Autodesk Inventor part; units mm, degrees
(part 3 of 4)
  line L513 (170.4618, 600.3596) -> (170.0567, 600.3596)
  line L514 (170.0567, 600.3596) -> (170.0567, 603.4076)
  line L515 (170.0567, 603.4076) -> (170.4618, 603.4076)
  line L516 (170.4618, 603.4076) -> (170.4618, 602.2121)
  line L517 (170.4618, 602.2121) -> (171.8647, 602.2121)
  line L518 (171.8647, 602.2121) -> (171.8647, 603.4076)
  line L519 (171.8647, 603.4076) -> (172.2698, 603.4076)
  line L520 (172.2698, 603.4076) -> (172.2698, 600.3596)
  line L521 (174.7621, 601.4069) -> (174.399, 601.4069)
  line L522 (174.399, 601.4069) -> (174.399, 600.3596)
  line L523 (174.399, 600.3596) -> (174.0063, 600.3596)
  line L524 (174.0063, 600.3596) -> (174.0063, 601.4069)
  line L525 (174.0063, 601.4069) -> (172.6601, 601.4069)
  line L526 (172.6601, 601.4069) -> (172.6601, 601.8366)
  line L527 (172.6601, 601.8366) -> (174.0235, 603.4076)
  line L528 (174.0235, 603.4076) -> (174.399, 603.4076)
  line L529 (174.399, 603.4076) -> (174.399, 601.7354)
  line L530 (174.399, 601.7354) -> (174.7621, 601.7354)
  line L531 (174.7621, 601.7354) -> (174.7621, 601.4069)
  line L532 (174.0063, 601.7354) -> (174.0063, 602.9259)
  line L533 (174.0063, 602.9259) -> (172.9812, 601.7354)
  line L534 (172.9812, 601.7354) -> (174.0063, 601.7354)
  line L535 (176.9678, 600.3596) -> (175.0881, 600.3596)
  line L536 (175.0881, 600.3596) -> (175.0881, 600.7918)
  spline S514 degree 2 poles (175.0881, 600.7918) (175.2907, 600.982) (175.6513, 601.3352) (175.8242, 601.5254) knots 0 0 0 1 2 2 2
  spline S515 degree 2 poles (175.8242, 601.5254) (176.1725, 601.9083) (176.4269, 602.3677) (176.4269, 602.6122) knots 0 0 0 1 2 2 2
  spline S516 degree 2 poles (176.4269, 602.6122) (176.4269, 602.7407) (176.3478, 602.9333) (176.2762, 602.9951) knots 0 0 0 1 2 2 2
  spline S517 degree 2 poles (176.2762, 602.9951) (176.2046, 603.0568) (176.0168, 603.1186) (175.9032, 603.1186) knots 0 0 0 1 2 2 2
  spline S518 degree 2 poles (175.9032, 603.1186) (175.7945, 603.1186) (175.5722, 603.0642) (175.471, 603.0222) knots 0 0 0 1 2 2 2
  spline S519 degree 2 poles (175.471, 603.0222) (175.3845, 602.9877) (175.224, 602.8889) (175.1746, 602.8543) knots 0 0 0 1 2 2 2
  line L537 (175.1746, 602.8543) -> (175.1523, 602.8543)
  line L538 (175.1523, 602.8543) -> (175.1523, 603.289)
  spline S520 degree 2 poles (175.1523, 603.289) (175.2783, 603.3508) (175.7303, 603.4718) (175.9329, 603.4718) knots 0 0 0 1 2 2 2
  spline S521 degree 2 poles (175.9329, 603.4718) (176.3602, 603.4718) (176.8418, 603.0198) (176.8418, 602.6344) knots 0 0 0 1 2 2 2
  spline S522 degree 2 poles (176.8418, 602.6344) (176.8418, 602.4541) (176.7578, 602.1528) (176.6837, 602.0244) knots 0 0 0 1 2 2 2
  spline S523 degree 2 poles (176.6837, 602.0244) (176.6096, 601.891) (176.3948, 601.6292) (176.2762, 601.5032) knots 0 0 0 1 2 2 2
  spline S524 degree 2 poles (176.2762, 601.5032) (176.0835, 601.2932) (175.6118, 600.8437) (175.471, 600.7128) knots 0 0 0 1 2 2 2
  line L539 (175.471, 600.7128) -> (176.9678, 600.7128)
  line L540 (176.9678, 600.7128) -> (176.9678, 600.3596)
  spline S525 degree 2 poles (179.3884, 602.4887) (179.3884, 602.2911) (179.2476, 601.9354) (179.1217, 601.8119) knots 0 0 0 1 2 2 2
  spline S526 degree 2 poles (179.1217, 601.8119) (178.9636, 601.6563) (178.5363, 601.4958) (178.2102, 601.4958) knots 0 0 0 1 2 2 2
  line L541 (178.2102, 601.4958) -> (177.8669, 601.4958)
  line L542 (177.8669, 601.4958) -> (177.8669, 600.3596)
  line L543 (177.8669, 600.3596) -> (177.4618, 600.3596)
  line L544 (177.4618, 600.3596) -> (177.4618, 603.4076)
  line L545 (177.4618, 603.4076) -> (178.2275, 603.4076)
  spline S527 degree 2 poles (178.2275, 603.4076) (178.4992, 603.4076) (178.8796, 603.3186) (179.0253, 603.2174) knots 0 0 0 1 2 2 2
  spline S528 degree 2 poles (179.0253, 603.2174) (179.1958, 603.1013) (179.3884, 602.7431) (179.3884, 602.4887) knots 0 0 0 1 2 2 2
  spline S529 degree 2 poles (178.966, 602.4764) (178.966, 602.6344) (178.8574, 602.8666) (178.7462, 602.9407) knots 0 0 0 1 2 2 2
  spline S530 degree 2 poles (178.7462, 602.9407) (178.6499, 603.005) (178.393, 603.0568) (178.2028, 603.0568) knots 0 0 0 1 2 2 2
  line L546 (178.2028, 603.0568) -> (177.8669, 603.0568)
  line L547 (177.8669, 603.0568) -> (177.8669, 601.8416)
  line L548 (177.8669, 601.8416) -> (178.1435, 601.8416)
  spline S531 degree 2 poles (178.1435, 601.8416) (178.3905, 601.8416) (178.6943, 601.9206) (178.7931, 602.0244) knots 0 0 0 1 2 2 2
  spline S532 degree 2 poles (178.7931, 602.0244) (178.8845, 602.1157) (178.966, 602.3306) (178.966, 602.4764) knots 0 0 0 1 2 2 2
  line L549 (181.9968, 600.3596) -> (181.4706, 600.3596)
  line L550 (181.4706, 600.3596) -> (180.3567, 601.7774)
  line L551 (180.3567, 601.7774) -> (180.1788, 601.5773)
  line L552 (180.1788, 601.5773) -> (180.1788, 600.3596)
  line L553 (180.1788, 600.3596) -> (179.7737, 600.3596)
  line L554 (179.7737, 600.3596) -> (179.7737, 603.4076)
  line L555 (179.7737, 603.4076) -> (180.1788, 603.4076)
  line L556 (180.1788, 603.4076) -> (180.1788, 602.0071)
  line L557 (180.1788, 602.0071) -> (181.4286, 603.4076)
  line L558 (181.4286, 603.4076) -> (181.9227, 603.4076)
  line L559 (181.9227, 603.4076) -> (180.6605, 602.0466)
  line L560 (180.6605, 602.0466) -> (181.9968, 600.3596)
  line L561 (183.4195, 603.5434) -> (182.2265, 599.6976)
  line L562 (182.2265, 599.6976) -> (181.8807, 599.6976)
  line L563 (181.8807, 599.6976) -> (183.0687, 603.5434)
  line L564 (183.0687, 603.5434) -> (183.4195, 603.5434)
  line L565 (185.025, 602.2343) -> (185.0052, 602.2343)
  spline S533 degree 2 poles (185.0052, 602.2343) (184.9608, 602.2467) (184.8644, 602.2516) (184.7978, 602.2516) knots 0 0 0 1 2 2 2
  spline S534 degree 2 poles (184.7978, 602.2516) (184.6421, 602.2516) (184.3359, 602.1157) (184.1975, 601.9824) knots 0 0 0 1 2 2 2
  line L566 (184.1975, 601.9824) -> (184.1975, 600.3596)
  line L567 (184.1975, 600.3596) -> (183.8122, 600.3596)
  line L568 (183.8122, 600.3596) -> (183.8122, 602.6468)
  line L569 (183.8122, 602.6468) -> (184.1975, 602.6468)
  line L570 (184.1975, 602.6468) -> (184.1975, 602.3059)
  spline S535 degree 2 poles (184.1975, 602.3059) (184.4075, 602.4937) (184.7212, 602.6468) (184.8694, 602.6468) knots 0 0 0 1 2 2 2
  spline S536 degree 2 poles (184.8694, 602.6468) (184.9287, 602.6468) (184.9879, 602.6419) (185.025, 602.6344) knots 0 0 0 1 2 2 2
  line L571 (185.025, 602.6344) -> (185.025, 602.2343)
  spline S537 degree 2 poles (186.3168, 600.3077) (185.7685, 600.3077) (185.1658, 600.9227) (185.1658, 601.4908) knots 0 0 0 1 2 2 2
  spline S538 degree 2 poles (185.1658, 601.4908) (185.1658, 602.0491) (185.7512, 602.711) (186.223, 602.711) knots 0 0 0 1 2 2 2
  spline S539 degree 2 poles (186.223, 602.711) (186.4354, 602.711) (186.7639, 602.5875) (186.8849, 602.4566) knots 0 0 0 1 2 2 2
  spline S540 degree 2 poles (186.8849, 602.4566) (187.0084, 602.3257) (187.1393, 601.9478) (187.1393, 601.6736) knots 0 0 0 1 2 2 2
  line L572 (187.1393, 601.6736) -> (187.1393, 601.4637)
  line L573 (187.1393, 601.4637) -> (185.556, 601.4637)
  spline S541 degree 2 poles (185.556, 601.4637) (185.556, 601.066) (185.9562, 600.6436) (186.3119, 600.6436) knots 0 0 0 1 2 2 2
  spline S542 degree 2 poles (186.3119, 600.6436) (186.4378, 600.6436) (186.6824, 600.7004) (186.7812, 600.7449) knots 0 0 0 1 2 2 2
  spline S543 degree 2 poles (186.7812, 600.7449) (186.8849, 600.7943) (187.0282, 600.8807) (187.0751, 600.9203) knots 0 0 0 1 2 2 2
  line L574 (187.0751, 600.9203) -> (187.0973, 600.9203)
  line L575 (187.0973, 600.9203) -> (187.0973, 600.5004)
  spline S544 degree 2 poles (187.0973, 600.5004) (187.0306, 600.4732) (186.8281, 600.3941) (186.7491, 600.3719) knots 0 0 0 1 2 2 2
  spline S545 degree 2 poles (186.7491, 600.3719) (186.6379, 600.3398) (186.4551, 600.3077) (186.3168, 600.3077) knots 0 0 0 1 2 2 2
  spline S546 degree 2 poles (186.7639, 601.7576) (186.7589, 601.9132) (186.6947, 602.1404) (186.633, 602.217) knots 0 0 0 1 2 2 2
  spline S547 degree 2 poles (186.633, 602.217) (186.5663, 602.3035) (186.3563, 602.3949) (186.2007, 602.3949) knots 0 0 0 1 2 2 2
  spline S548 degree 2 poles (186.2007, 602.3949) (186.0476, 602.3949) (185.8327, 602.3035) (185.7438, 602.2145) knots 0 0 0 1 2 2 2
  spline S549 degree 2 poles (185.7438, 602.2145) (185.6573, 602.1232) (185.5684, 601.9033) (185.556, 601.7576) knots 0 0 0 1 2 2 2
  line L576 (185.556, 601.7576) -> (186.7639, 601.7576)
  line L577 (188.7325, 603.1729) -> (188.7127, 603.1729)
  spline S550 degree 2 poles (188.7127, 603.1729) (188.6609, 603.1927) (188.4682, 603.2273) (188.3916, 603.2273) knots 0 0 0 1 2 2 2
  spline S551 degree 2 poles (188.3916, 603.2273) (188.1496, 603.2273) (187.9421, 603.0099) (187.9421, 602.7234) knots 0 0 0 1 2 2 2
  line L578 (187.9421, 602.7234) -> (187.9421, 602.6468)
  line L579 (187.9421, 602.6468) -> (188.5793, 602.6468)
  line L580 (188.5793, 602.6468) -> (188.5793, 602.3282)
  line L581 (188.5793, 602.3282) -> (187.9544, 602.3282)
  line L582 (187.9544, 602.3282) -> (187.9544, 600.3596)
  line L583 (187.9544, 600.3596) -> (187.5691, 600.3596)
  line L584 (187.5691, 600.3596) -> (187.5691, 602.3282)
  line L585 (187.5691, 602.3282) -> (187.3098, 602.3282)
  line L586 (187.3098, 602.3282) -> (187.3098, 602.6468)
  line L587 (187.3098, 602.6468) -> (187.5691, 602.6468)
  line L588 (187.5691, 602.6468) -> (187.5691, 602.7234)
  spline S552 degree 2 poles (187.5691, 602.7234) (187.5691, 603.1334) (187.9668, 603.5632) (188.3373, 603.5632) knots 0 0 0 1 2 2 2
  spline S553 degree 2 poles (188.3373, 603.5632) (188.4435, 603.5632) (188.6485, 603.5409) (188.7325, 603.5261) knots 0 0 0 1 2 2 2
  line L589 (188.7325, 603.5261) -> (188.7325, 603.1729)
  line L590 (191.2396, 601.1006) -> (188.977, 601.1006)
  line L591 (188.977, 601.1006) -> (188.977, 601.4291)
  line L592 (188.977, 601.4291) -> (191.2396, 601.4291)
  line L593 (191.2396, 601.4291) -> (191.2396, 601.1006)
  line L594 (191.2396, 601.9601) -> (188.977, 601.9601)
  line L595 (188.977, 601.9601) -> (188.977, 602.2886)
  line L596 (188.977, 602.2886) -> (191.2396, 602.2886)
  line L597 (191.2396, 602.2886) -> (191.2396, 601.9601)
  spline S554 degree 2 poles (192.5314, 600.3052) (192.3017, 600.3052) (191.904, 600.4287) (191.7731, 600.4979) knots 0 0 0 1 2 2 2
  line L598 (191.7731, 600.4979) -> (191.7731, 600.9301)
  line L599 (191.7731, 600.9301) -> (191.7928, 600.9301)
  spline S555 degree 2 poles (191.7928, 600.9301) (191.8422, 600.8906) (191.9756, 600.7968) (192.0868, 600.7449) knots 0 0 0 1 2 2 2
  spline S556 degree 2 poles (192.0868, 600.7449) (192.1831, 600.698) (192.4202, 600.6288) (192.5462, 600.6288) knots 0 0 0 1 2 2 2
  spline S557 degree 2 poles (192.5462, 600.6288) (192.6376, 600.6288) (192.8475, 600.6708) (192.8969, 600.7054) knots 0 0 0 1 2 2 2
  spline S558 degree 2 poles (192.8969, 600.7054) (192.9686, 600.7523) (193.0328, 600.8585) (193.0328, 600.9672) knots 0 0 0 1 2 2 2
  spline S559 degree 2 poles (193.0328, 600.9672) (193.0328, 601.103) (192.8846, 601.2438) (192.6944, 601.2908) knots 0 0 0 1 2 2 2
  spline S560 degree 2 poles (192.6944, 601.2908) (192.6203, 601.3081) (192.3832, 601.3575) (192.2819, 601.3846) knots 0 0 0 1 2 2 2
  spline S561 degree 2 poles (192.2819, 601.3846) (192.0201, 601.4612) (191.783, 601.7774) (191.783, 602.0021) knots 0 0 0 1 2 2 2
  spline S562 degree 2 poles (191.783, 602.0021) (191.783, 602.3133) (192.2498, 602.7011) (192.6351, 602.7011) knots 0 0 0 1 2 2 2
  spline S563 degree 2 poles (192.6351, 602.7011) (192.8253, 602.7011) (193.2106, 602.6073) (193.3415, 602.5356) knots 0 0 0 1 2 2 2
  line L600 (193.3415, 602.5356) -> (193.3415, 602.1232)
  line L601 (193.3415, 602.1232) -> (193.3218, 602.1232)
  spline S564 degree 2 poles (193.3218, 602.1232) (193.1736, 602.2417) (192.813, 602.3776) (192.6277, 602.3776) knots 0 0 0 1 2 2 2
  spline S565 degree 2 poles (192.6277, 602.3776) (192.4375, 602.3776) (192.1757, 602.217) (192.1757, 602.0565) knots 0 0 0 1 2 2 2
  spline S566 degree 2 poles (192.1757, 602.0565) (192.1757, 601.9107) (192.3313, 601.7699) (192.5042, 601.7255) knots 0 0 0 1 2 2 2
  spline S567 degree 2 poles (192.5042, 601.7255) (192.5882, 601.7033) (192.8006, 601.6588) (192.9167, 601.6316) knots 0 0 0 1 2 2 2
  spline S568 degree 2 poles (192.9167, 601.6316) (193.1686, 601.5674) (193.4255, 601.2735) (193.4255, 601.0191) knots 0 0 0 1 2 2 2
  spline S569 degree 2 poles (193.4255, 601.0191) (193.4255, 600.8709) (193.3094, 600.609) (193.1958, 600.5127) knots 0 0 0 1 2 2 2
  spline S570 degree 2 poles (193.1958, 600.5127) (193.0748, 600.4114) (192.766, 600.3052) (192.5314, 600.3052) knots 0 0 0 1 2 2 2
  line L602 (194.9964, 602.2343) -> (194.9767, 602.2343)
  spline S571 degree 2 poles (194.9767, 602.2343) (194.9322, 602.2467) (194.8359, 602.2516) (194.7692, 602.2516) knots 0 0 0 1 2 2 2
  spline S572 degree 2 poles (194.7692, 602.2516) (194.6136, 602.2516) (194.3073, 602.1157) (194.169, 601.9824) knots 0 0 0 1 2 2 2
  line L603 (194.169, 601.9824) -> (194.169, 600.3596)
  line L604 (194.169, 600.3596) -> (193.7837, 600.3596)
  line L605 (193.7837, 600.3596) -> (193.7837, 602.6468)
  line L606 (193.7837, 602.6468) -> (194.169, 602.6468)
  line L607 (194.169, 602.6468) -> (194.169, 602.3059)
  spline S573 degree 2 poles (194.169, 602.3059) (194.3789, 602.4937) (194.6926, 602.6468) (194.8408, 602.6468) knots 0 0 0 1 2 2 2
  spline S574 degree 2 poles (194.8408, 602.6468) (194.9001, 602.6468) (194.9594, 602.6419) (194.9964, 602.6344) knots 0 0 0 1 2 2 2
  line L608 (194.9964, 602.6344) -> (194.9964, 602.2343)
  line L609 (197.3356, 599.747) -> (194.9841, 599.747)
  line L610 (194.9841, 599.747) -> (194.9841, 600.0113)
  line L611 (194.9841, 600.0113) -> (197.3356, 600.0113)
  line L612 (197.3356, 600.0113) -> (197.3356, 599.747)
  line L613 (199.2523, 600.3596) -> (197.7653, 600.3596)
  line L614 (197.7653, 600.3596) -> (197.7653, 600.6708)
  line L615 (197.7653, 600.6708) -> (198.3186, 600.6708)
  line L616 (198.3186, 600.6708) -> (198.3186, 602.7135)
  line L617 (198.3186, 602.7135) -> (197.7653, 602.7135)
  line L618 (197.7653, 602.7135) -> (197.7653, 602.9926)
  spline S575 degree 2 poles (197.7653, 602.9926) (198.079, 602.9926) (198.3754, 603.1704) (198.3952, 603.4174) knots 0 0 0 1 2 2 2
  line L619 (198.3952, 603.4174) -> (198.7114, 603.4174)
  line L620 (198.7114, 603.4174) -> (198.7114, 600.6708)
  line L621 (198.7114, 600.6708) -> (199.2523, 600.6708)
  line L622 (199.2523, 600.6708) -> (199.2523, 600.3596)
  line L623 (201.91, 599.747) -> (199.5586, 599.747)
  line L624 (199.5586, 599.747) -> (199.5586, 600.0113)
  line L625 (199.5586, 600.0113) -> (201.91, 600.0113)
  line L626 (201.91, 600.0113) -> (201.91, 599.747)
  spline S576 degree 2 poles (202.9227, 603.1186) (202.8116, 603.1186) (202.5917, 603.0642) (202.4855, 603.0222) knots 0 0 0 1 2 2 2
  spline S577 degree 2 poles (202.4855, 603.0222) (202.3867, 602.9803) (202.241, 602.8913) (202.1842, 602.8518) knots 0 0 0 1 2 2 2
  line L627 (202.1842, 602.8518) -> (202.1595, 602.8518)
  line L628 (202.1595, 602.8518) -> (202.1595, 603.2841)
  spline S578 degree 2 poles (202.1595, 603.2841) (202.2929, 603.3557) (202.7498, 603.4718) (202.9548, 603.4718) knots 0 0 0 1 2 2 2
  spline S579 degree 2 poles (202.9548, 603.4718) (203.1623, 603.4718) (203.4711, 603.3878) (203.597, 603.2989) knots 0 0 0 1 2 2 2
  spline S580 degree 2 poles (203.597, 603.2989) (203.7304, 603.2026) (203.8687, 602.9234) (203.8687, 602.7357) knots 0 0 0 1 2 2 2
  spline S581 degree 2 poles (203.8687, 602.7357) (203.8687, 602.4838) (203.5378, 602.1034) (203.3056, 602.054) knots 0 0 0 1 2 2 2
  line L629 (203.3056, 602.054) -> (203.3056, 602.0244)
  spline S582 degree 2 poles (203.3056, 602.0244) (203.4019, 602.0046) (203.6217, 601.9157) (203.7156, 601.8268) knots 0 0 0 1 2 2 2
  spline S583 degree 2 poles (203.7156, 601.8268) (203.8095, 601.7403) (203.928, 601.4637) (203.928, 601.2636) knots 0 0 0 1 2 2 2
  spline S584 degree 2 poles (203.928, 601.2636) (203.928, 601.0586) (203.7872, 600.7103) (203.6588, 600.5769) knots 0 0 0 1 2 2 2
  spline S585 degree 2 poles (203.6588, 600.5769) (203.5254, 600.4386) (203.1475, 600.2953) (202.9079, 600.2953) knots 0 0 0 1 2 2 2
  spline S586 degree 2 poles (202.9079, 600.2953) (202.6782, 600.2953) (202.2287, 600.4065) (202.0755, 600.4831) knots 0 0 0 1 2 2 2
  line L630 (202.0755, 600.4831) -> (202.0755, 600.9153)
  line L631 (202.0755, 600.9153) -> (202.1052, 600.9153)
  spline S587 degree 2 poles (202.1052, 600.9153) (202.2336, 600.8215) (202.6683, 600.6486) (202.8832, 600.6486) knots 0 0 0 1 2 2 2
  spline S588 degree 2 poles (202.8832, 600.6486) (203.0092, 600.6486) (203.2611, 600.7276) (203.3451, 600.819) knots 0 0 0 1 2 2 2
  spline S589 degree 2 poles (203.3451, 600.819) (203.4266, 600.9104) (203.5131, 601.1277) (203.5131, 601.2932) knots 0 0 0 1 2 2 2
  spline S590 degree 2 poles (203.5131, 601.2932) (203.5131, 601.4587) (203.4167, 601.6736) (203.3303, 601.7354) knots 0 0 0 1 2 2 2
  spline S591 degree 2 poles (203.3303, 601.7354) (203.2438, 601.7971) (203.0092, 601.844) (202.8709, 601.844) knots 0 0 0 1 2 2 2
  line L632 (202.8709, 601.844) -> (202.698, 601.844)
  line L633 (202.698, 601.844) -> (202.698, 602.1824)
  line L634 (202.698, 602.1824) -> (202.8338, 602.1824)
  spline S592 degree 2 poles (202.8338, 602.1824) (203.108, 602.1824) (203.4538, 602.4443) (203.4538, 602.6937) knots 0 0 0 1 2 2 2
  spline S593 degree 2 poles (203.4538, 602.6937) (203.4538, 602.8098) (203.3649, 602.9753) (203.2932, 603.0247) knots 0 0 0 1 2 2 2
  spline S594 degree 2 poles (203.2932, 603.0247) (203.2167, 603.0766) (203.0289, 603.1186) (202.9227, 603.1186) knots 0 0 0 1 2 2 2
  spline S595 degree 2 poles (206.03, 602.6913) (206.03, 602.4912) (205.8966, 602.1775) (205.7855, 602.0589) knots 0 0 0 1 2 2 2
  spline S596 degree 2 poles (205.7855, 602.0589) (205.6768, 601.9404) (205.3952, 601.7403) (205.2396, 601.6464) knots 0 0 0 1 2 2 2
  line L635 (205.2396, 601.6464) -> (205.2396, 601.1796)
  line L636 (205.2396, 601.1796) -> (204.874, 601.1796)
  line L637 (204.874, 601.1796) -> (204.874, 601.8045)
  spline S597 degree 2 poles (204.874, 601.8045) (204.9877, 601.8737) (205.2939, 602.0663) (205.3804, 602.1503) knots 0 0 0 1 2 2 2
  spline S598 degree 2 poles (205.3804, 602.1503) (205.4891, 602.2565) (205.6126, 602.5035) (205.6126, 602.6616) knots 0 0 0 1 2 2 2
  spline S599 degree 2 poles (205.6126, 602.6616) (205.6126, 602.8913) (205.3211, 603.1186) (205.0889, 603.1186) knots 0 0 0 1 2 2 2
  spline S600 degree 2 poles (205.0889, 603.1186) (204.8839, 603.1186) (204.5233, 602.9827) (204.4097, 602.9086) knots 0 0 0 1 2 2 2
  line L638 (204.4097, 602.9086) -> (204.3875, 602.9086)
  line L639 (204.3875, 602.9086) -> (204.3875, 603.3261)
  spline S601 degree 2 poles (204.3875, 603.3261) (204.5233, 603.3804) (204.9407, 603.4693) (205.1285, 603.4693) knots 0 0 0 1 2 2 2
  spline S602 degree 2 poles (205.1285, 603.4693) (205.5484, 603.4693) (206.03, 603.042) (206.03, 602.6913) knots 0 0 0 1 2 2 2
  line L640 (205.2717, 600.3596) -> (204.8568, 600.3596)
  line L641 (204.8568, 600.3596) -> (204.8568, 600.7918)
  line L642 (204.8568, 600.7918) -> (205.2717, 600.7918)
  line L643 (205.2717, 600.7918) -> (205.2717, 600.3596)
  line L644 (206.8229, 600.3596) -> (206.4376, 600.3596)
  line L645 (206.4376, 600.3596) -> (206.4376, 602.6468)
  line L646 (206.4376, 602.6468) -> (206.8229, 602.6468)
  line L647 (206.8229, 602.6468) -> (206.8229, 600.3596)
  line L648 (206.8501, 603.0272) -> (206.4129, 603.0272)
  line L649 (206.4129, 603.0272) -> (206.4129, 603.4273)
  line L650 (206.4129, 603.4273) -> (206.8501, 603.4273)
  line L651 (206.8501, 603.4273) -> (206.8501, 603.0272)
  spline S603 degree 2 poles (208.3815, 600.3077) (207.8331, 600.3077) (207.2304, 600.9227) (207.2304, 601.4908) knots 0 0 0 1 2 2 2
  spline S604 degree 2 poles (207.2304, 601.4908) (207.2304, 602.0491) (207.8158, 602.711) (208.2876, 602.711) knots 0 0 0 1 2 2 2
  spline S605 degree 2 poles (208.2876, 602.711) (208.5, 602.711) (208.8285, 602.5875) (208.9496, 602.4566) knots 0 0 0 1 2 2 2
  spline S606 degree 2 poles (208.9496, 602.4566) (209.0731, 602.3257) (209.204, 601.9478) (209.204, 601.6736) knots 0 0 0 1 2 2 2
  line L652 (209.204, 601.6736) -> (209.204, 601.4637)
  line L653 (209.204, 601.4637) -> (207.6207, 601.4637)
  spline S607 degree 2 poles (207.6207, 601.4637) (207.6207, 601.066) (208.0208, 600.6436) (208.3765, 600.6436) knots 0 0 0 1 2 2 2
  spline S608 degree 2 poles (208.3765, 600.6436) (208.5025, 600.6436) (208.747, 600.7004) (208.8458, 600.7449) knots 0 0 0 1 2 2 2
  spline S609 degree 2 poles (208.8458, 600.7449) (208.9496, 600.7943) (209.0928, 600.8807) (209.1398, 600.9203) knots 0 0 0 1 2 2 2
  line L654 (209.1398, 600.9203) -> (209.162, 600.9203)
  line L655 (209.162, 600.9203) -> (209.162, 600.5004)
  spline S610 degree 2 poles (209.162, 600.5004) (209.0953, 600.4732) (208.8928, 600.3941) (208.8137, 600.3719) knots 0 0 0 1 2 2 2
  spline S611 degree 2 poles (208.8137, 600.3719) (208.7026, 600.3398) (208.5198, 600.3077) (208.3815, 600.3077) knots 0 0 0 1 2 2 2
  spline S612 degree 2 poles (208.8285, 601.7576) (208.8236, 601.9132) (208.7594, 602.1404) (208.6976, 602.217) knots 0 0 0 1 2 2 2
  spline S613 degree 2 poles (208.6976, 602.217) (208.6309, 602.3035) (208.421, 602.3949) (208.2654, 602.3949) knots 0 0 0 1 2 2 2
  spline S614 degree 2 poles (208.2654, 602.3949) (208.1122, 602.3949) (207.8973, 602.3035) (207.8084, 602.2145) knots 0 0 0 1 2 2 2
  spline S615 degree 2 poles (207.8084, 602.2145) (207.722, 602.1232) (207.6331, 601.9033) (207.6207, 601.7576) knots 0 0 0 1 2 2 2
  line L656 (207.6207, 601.7576) -> (208.8285, 601.7576)
  line L657 (211.9704, 601.1006) -> (209.7079, 601.1006)
  line L658 (209.7079, 601.1006) -> (209.7079, 601.4291)
  line L659 (209.7079, 601.4291) -> (211.9704, 601.4291)
  line L660 (211.9704, 601.4291) -> (211.9704, 601.1006)
  line L661 (211.9704, 601.9601) -> (209.7079, 601.9601)
  line L662 (209.7079, 601.9601) -> (209.7079, 602.2886)
  line L663 (209.7079, 602.2886) -> (211.9704, 602.2886)
  line L664 (211.9704, 602.2886) -> (211.9704, 601.9601)
  spline S616 degree 2 poles (213.7389, 600.2953) (213.4697, 600.2953) (213.0696, 600.4361) (212.9288, 600.5769) knots 0 0 0 1 2 2 2
  spline S617 degree 2 poles (212.9288, 600.5769) (212.7682, 600.735) (212.6373, 601.1796) (212.6373, 601.5057) knots 0 0 0 1 2 2 2
  line L665 (212.6373, 601.5057) -> (212.6373, 603.4076)
  line L666 (212.6373, 603.4076) -> (213.0424, 603.4076)
  line L667 (213.0424, 603.4076) -> (213.0424, 601.5057)
  spline S618 degree 2 poles (213.0424, 601.5057) (213.0424, 601.2932) (213.0967, 601.0067) (213.1733, 600.8906) knots 0 0 0 1 2 2 2
  spline S619 degree 2 poles (213.1733, 600.8906) (213.2548, 600.7671) (213.5364, 600.6411) (213.7389, 600.6411) knots 0 0 0 1 2 2 2
  spline S620 degree 2 poles (213.7389, 600.6411) (213.9291, 600.6411) (214.2255, 600.7671) (214.307, 600.8906) knots 0 0 0 1 2 2 2
  spline S621 degree 2 poles (214.307, 600.8906) (214.3836, 601.0067) (214.4379, 601.2908) (214.4379, 601.4958) knots 0 0 0 1 2 2 2
  line L668 (214.4379, 601.4958) -> (214.4379, 603.4076)
  line L669 (214.4379, 603.4076) -> (214.843, 603.4076)
  line L670 (214.843, 603.4076) -> (214.843, 601.5057)
  spline S622 degree 2 poles (214.843, 601.5057) (214.843, 601.187) (214.7146, 600.7325) (214.5516, 600.5769) knots 0 0 0 1 2 2 2
  spline S623 degree 2 poles (214.5516, 600.5769) (214.4058, 600.4337) (214.0205, 600.2953) (213.7389, 600.2953) knots 0 0 0 1 2 2 2
  line L671 (216.1348, 600.3596) -> (216.1348, 603.0469)
  line L672 (216.1348, 603.0469) -> (215.1123, 603.0469)
  line L673 (215.1123, 603.0469) -> (215.1123, 603.4076)
  line L674 (215.1123, 603.4076) -> (217.5625, 603.4076)
  line L675 (217.5625, 603.4076) -> (217.5625, 603.0469)
  line L676 (217.5625, 603.0469) -> (216.5399, 603.0469)
  line L677 (216.5399, 603.0469) -> (216.5399, 600.3596)
  line L678 (216.5399, 600.3596) -> (216.1348, 600.3596)
  line L679 (219.6941, 603.0469) -> (218.2764, 603.0469)
  line L680 (218.2764, 603.0469) -> (218.2764, 602.1874)
  line L681 (218.2764, 602.1874) -> (219.6349, 602.1874)
  line L682 (219.6349, 602.1874) -> (219.6349, 601.8268)
  line L683 (219.6349, 601.8268) -> (218.2764, 601.8268)
  line L684 (218.2764, 601.8268) -> (218.2764, 600.3596)
  line L685 (218.2764, 600.3596) -> (217.8713, 600.3596)
  line L686 (217.8713, 600.3596) -> (217.8713, 603.4076)
  line L687 (217.8713, 603.4076) -> (219.6941, 603.4076)
  line L688 (219.6941, 603.4076) -> (219.6941, 603.0469)
  spline S624 degree 2 poles (220.8921, 600.2904) (220.6649, 600.2904) (220.2919, 600.4263) (220.161, 600.5522) knots 0 0 0 1 2 2 2
  spline S625 degree 2 poles (220.161, 600.5522) (220.0325, 600.6757) (219.8992, 601.0116) (219.8992, 601.2018) knots 0 0 0 1 2 2 2
  spline S626 degree 2 poles (219.8992, 601.2018) (219.8992, 601.4488) (220.1634, 601.8638) (220.4154, 601.9873) knots 0 0 0 1 2 2 2
  line L689 (220.4154, 601.9873) -> (220.4154, 601.9997)
  spline S627 degree 2 poles (220.4154, 601.9997) (220.1906, 602.1306) (219.9733, 602.4418) (219.9733, 602.674) knots 0 0 0 1 2 2 2
  spline S628 degree 2 poles (219.9733, 602.674) (219.9733, 603.0173) (220.492, 603.4767) (220.8921, 603.4767) knots 0 0 0 1 2 2 2
  spline S629 degree 2 poles (220.8921, 603.4767) (221.3071, 603.4767) (221.8085, 603.042) (221.8085, 602.7011) knots 0 0 0 1 2 2 2
  spline S630 degree 2 poles (221.8085, 602.7011) (221.8085, 602.4961) (221.5689, 602.096) (221.3441, 601.9824) knots 0 0 0 1 2 2 2
  line L690 (221.3441, 601.9824) -> (221.3441, 601.97)
  spline S631 degree 2 poles (221.3441, 601.97) (221.6109, 601.8465) (221.885, 601.4908) (221.885, 601.2093) knots 0 0 0 1 2 2 2
  spline S632 degree 2 poles (221.885, 601.2093) (221.885, 600.819) (221.3169, 600.2904) (220.8921, 600.2904) knots 0 0 0 1 2 2 2
  spline S633 degree 2 poles (221.4651, 601.1697) (221.4651, 601.3575) (221.3169, 601.5798) (221.107, 601.6934) knots 0 0 0 1 2 2 2
  spline S634 degree 2 poles (221.107, 601.6934) (221.0378, 601.7329) (220.8056, 601.8243) (220.6599, 601.8836) knots 0 0 0 1 2 2 2
  spline S635 degree 2 poles (220.6599, 601.8836) (220.492, 601.7724) (220.3116, 601.4414) (220.3116, 601.2315) knots 0 0 0 1 2 2 2
  spline S636 degree 2 poles (220.3116, 601.2315) (220.3116, 600.9548) (220.6451, 600.5942) (220.897, 600.5942) knots 0 0 0 1 2 2 2
  spline S637 degree 2 poles (220.897, 600.5942) (221.1539, 600.5942) (221.4651, 600.903) (221.4651, 601.1697) knots 0 0 0 1 2 2 2
  spline S638 degree 2 poles (221.4083, 602.6962) (221.4083, 602.9012) (221.1342, 603.1754) (220.8896, 603.1754) knots 0 0 0 1 2 2 2
  spline S639 degree 2 poles (220.8896, 603.1754) (220.6673, 603.1754) (220.3833, 602.9309) (220.3833, 602.7209) knots 0 0 0 1 2 2 2
  spline S640 degree 2 poles (220.3833, 602.7209) (220.3833, 602.5702) (220.529, 602.3603) (220.6747, 602.2763) knots 0 0 0 1 2 2 2
  spline S641 degree 2 poles (220.6747, 602.2763) (220.7365, 602.2417) (220.9983, 602.1207) (221.1045, 602.0861) knots 0 0 0 1 2 2 2
  spline S642 degree 2 poles (221.1045, 602.0861) (221.2824, 602.222) (221.4083, 602.5109) (221.4083, 602.6962) knots 0 0 0 1 2 2 2
  line L691 (224.9923, 600.3596) -> (224.4687, 600.3596)
  line L692 (224.4687, 600.3596) -> (224.0512, 600.7968)
  spline S643 degree 2 poles (224.0512, 600.7968) (223.8438, 600.53) (223.4041, 600.2953) (223.125, 600.2953) knots 0 0 0 1 2 2 2
  spline S644 degree 2 poles (223.125, 600.2953) (222.7125, 600.2953) (222.174, 600.7943) (222.174, 601.1969) knots 0 0 0 1 2 2 2
  spline S645 degree 2 poles (222.174, 601.1969) (222.174, 601.3723) (222.2728, 601.6464) (222.3543, 601.7576) knots 0 0 0 1 2 2 2
  spline S646 degree 2 poles (222.3543, 601.7576) (222.4334, 601.8638) (222.6433, 602.0268) (222.7372, 602.0861) knots 0 0 0 1 2 2 2
  spline S647 degree 2 poles (222.7372, 602.0861) (222.5322, 602.2244) (222.3272, 602.5332) (222.3272, 602.7654) knots 0 0 0 1 2 2 2
  spline S648 degree 2 poles (222.3272, 602.7654) (222.3272, 602.9111) (222.4433, 603.1581) (222.5371, 603.252) knots 0 0 0 1 2 2 2
  spline S649 degree 2 poles (222.5371, 603.252) (222.6359, 603.3483) (222.9496, 603.4718) (223.1349, 603.4718) knots 0 0 0 1 2 2 2
  spline S650 degree 2 poles (223.1349, 603.4718) (223.4757, 603.4718) (223.9055, 603.1136) (223.9055, 602.8395) knots 0 0 0 1 2 2 2
  spline S651 degree 2 poles (223.9055, 602.8395) (223.9055, 602.7382) (223.8536, 602.5233) (223.787, 602.4245) knots 0 0 0 1 2 2 2
  spline S652 degree 2 poles (223.787, 602.4245) (223.7178, 602.3232) (223.5004, 602.1479) (223.3177, 602.0812) knots 0 0 0 1 2 2 2
  line L693 (223.3177, 602.0812) -> (224.0364, 601.3402)
  spline S653 degree 2 poles (224.0364, 601.3402) (224.0636, 601.5081) (224.0759, 601.9033) (224.0759, 602.222) knots 0 0 0 1 2 2 2
  line L694 (224.0759, 602.222) -> (224.4761, 602.222)
  line L695 (224.4761, 602.222) -> (224.4761, 602.0244)
  spline S654 degree 2 poles (224.4761, 602.0244) (224.4761, 601.8292) (224.3773, 601.3352) (224.2612, 601.1129) knots 0 0 0 1 2 2 2
  line L696 (224.2612, 601.1129) -> (224.9923, 600.3596)
  line L697 (223.8734, 600.9771) -> (222.9323, 601.9404)
  spline S655 degree 2 poles (222.9323, 601.9404) (222.8829, 601.9083) (222.7817, 601.8169) (222.7199, 601.728) knots 0 0 0 1 2 2 2
  spline S656 degree 2 poles (222.7199, 601.728) (222.6705, 601.6563) (222.5964, 601.4241) (222.5964, 601.2957) knots 0 0 0 1 2 2 2
  spline S657 degree 2 poles (222.5964, 601.2957) (222.5964, 601.0042) (222.9422, 600.6288) (223.2361, 600.6288) knots 0 0 0 1 2 2 2
  spline S658 degree 2 poles (223.2361, 600.6288) (223.4313, 600.6288) (223.745, 600.7943) (223.8734, 600.9771) knots 0 0 0 1 2 2 2
  spline S659 degree 2 poles (223.125, 602.2269) (223.2386, 602.2664) (223.3893, 602.3973) (223.4313, 602.4739) knots 0 0 0 1 2 2 2
  spline S660 degree 2 poles (223.4313, 602.4739) (223.4683, 602.5455) (223.5054, 602.7061) (223.5054, 602.7999) knots 0 0 0 1 2 2 2
  spline S661 degree 2 poles (223.5054, 602.7999) (223.5054, 602.9975) (223.2732, 603.2149) (223.1201, 603.2149) knots 0 0 0 1 2 2 2
  spline S662 degree 2 poles (223.1201, 603.2149) (222.9373, 603.2149) (222.7273, 602.9679) (222.7273, 602.7851) knots 0 0 0 1 2 2 2
  spline S663 degree 2 poles (222.7273, 602.7851) (222.7273, 602.7036) (222.757, 602.585) (222.8064, 602.5085) knots 0 0 0 1 2 2 2
  spline S664 degree 2 poles (222.8064, 602.5085) (222.8508, 602.4443) (223.004, 602.301) (223.125, 602.2269) knots 0 0 0 1 2 2 2
  line L698 (226.8967, 599.5173) -> (226.5114, 599.5173)
  line L699 (226.5114, 599.5173) -> (226.5114, 600.609)
  spline S665 degree 2 poles (226.5114, 600.609) (226.3434, 600.4559) (226.0248, 600.3151) (225.8297, 600.3151) knots 0 0 0 1 2 2 2
  spline S666 degree 2 poles (225.8297, 600.3151) (225.4419, 600.3151) (224.98, 600.94) (224.98, 601.4958) knots 0 0 0 1 2 2 2
  spline S667 degree 2 poles (224.98, 601.4958) (224.98, 601.7922) (225.1405, 602.2442) (225.2739, 602.3973) knots 0 0 0 1 2 2 2
  spline S668 degree 2 poles (225.2739, 602.3973) (225.4023, 602.548) (225.7531, 602.711) (225.9433, 602.711) knots 0 0 0 1 2 2 2
  spline S669 degree 2 poles (225.9433, 602.711) (226.1187, 602.711) (226.3755, 602.6295) (226.5114, 602.548) knots 0 0 0 1 2 2 2
  line L700 (226.5114, 602.548) -> (226.5361, 602.6468)
  line L701 (226.5361, 602.6468) -> (226.8967, 602.6468)
  line L702 (226.8967, 602.6468) -> (226.8967, 599.5173)
  line L703 (226.5114, 600.9326) -> (226.5114, 602.2368)
  spline S670 degree 2 poles (226.5114, 602.2368) (226.3657, 602.3084) (226.1384, 602.3652) (226.0075, 602.3652) knots 0 0 0 1 2 2 2
  spline S671 degree 2 poles (226.0075, 602.3652) (225.7037, 602.3652) (225.3776, 601.9256) (225.3776, 601.5155) knots 0 0 0 1 2 2 2
  spline S672 degree 2 poles (225.3776, 601.5155) (225.3776, 601.1129) (225.6395, 600.6807) (225.9161, 600.6807) knots 0 0 0 1 2 2 2
  spline S673 degree 2 poles (225.9161, 600.6807) (226.0767, 600.6807) (226.3829, 600.819) (226.5114, 600.9326) knots 0 0 0 1 2 2 2
  line L704 (227.8477, 600.3596) -> (227.4623, 600.3596)
  line L705 (227.4623, 600.3596) -> (227.4623, 602.6468)
  line L706 (227.4623, 602.6468) -> (227.8477, 602.6468)
  line L707 (227.8477, 602.6468) -> (227.8477, 600.3596)
  line L708 (227.8748, 603.0272) -> (227.4376, 603.0272)
  line L709 (227.4376, 603.0272) -> (227.4376, 603.4273)
  line L710 (227.4376, 603.4273) -> (227.8748, 603.4273)
  line L711 (227.8748, 603.4273) -> (227.8748, 603.0272)
  line L712 (230.1719, 600.3596) -> (229.7866, 600.3596)
  line L713 (229.7866, 600.3596) -> (229.7866, 600.5917)
  spline S674 degree 2 poles (229.7866, 600.5917) (229.6977, 600.5176) (229.5668, 600.4188) (229.4779, 600.3769) knots 0 0 0 1 2 2 2
  spline S675 degree 2 poles (229.4779, 600.3769) (229.3964, 600.3373) (229.221, 600.2953) (229.1049, 600.2953) knots 0 0 0 1 2 2 2
  spline S676 degree 2 poles (229.1049, 600.2953) (228.9172, 600.2953) (228.601, 600.451) (228.4899, 600.6016) knots 0 0 0 1 2 2 2
  spline S677 degree 2 poles (228.4899, 600.6016) (228.3787, 600.7523) (228.2552, 601.1969) (228.2552, 601.4859) knots 0 0 0 1 2 2 2
  spline S678 degree 2 poles (228.2552, 601.4859) (228.2552, 601.7872) (228.4108, 602.2269) (228.5467, 602.3924) knots 0 0 0 1 2 2 2
  spline S679 degree 2 poles (228.5467, 602.3924) (228.6727, 602.5406) (229.0259, 602.711) (229.221, 602.711) knots 0 0 0 1 2 2 2
  spline S680 degree 2 poles (229.221, 602.711) (229.3914, 602.711) (229.6458, 602.6344) (229.7866, 602.5554) knots 0 0 0 1 2 2 2
  line L714 (229.7866, 602.5554) -> (229.7866, 603.5434)
  line L715 (229.7866, 603.5434) -> (230.1719, 603.5434)
  line L716 (230.1719, 603.5434) -> (230.1719, 600.3596)
  line L717 (229.7866, 600.9153) -> (229.7866, 602.2368)
  spline S681 degree 2 poles (229.7866, 602.2368) (229.6434, 602.3059) (229.4161, 602.3578) (229.2852, 602.3578) knots 0 0 0 1 2 2 2
  spline S682 degree 2 poles (229.2852, 602.3578) (228.9888, 602.3578) (228.6529, 601.9132) (228.6529, 601.4933) knots 0 0 0 1 2 2 2
  spline S683 degree 2 poles (228.6529, 601.4933) (228.6529, 601.0882) (228.9098, 600.6609) (229.1938, 600.6609) knots 0 0 0 1 2 2 2
  spline S684 degree 2 poles (229.1938, 600.6609) (229.3445, 600.6609) (229.6508, 600.7992) (229.7866, 600.9153) knots 0 0 0 1 2 2 2
  line L718 (233.1063, 601.1006) -> (230.8438, 601.1006)
  line L719 (230.8438, 601.1006) -> (230.8438, 601.4291)
  line L720 (230.8438, 601.4291) -> (233.1063, 601.4291)
  line L721 (233.1063, 601.4291) -> (233.1063, 601.1006)
  line L722 (233.1063, 601.9601) -> (230.8438, 601.9601)
  line L723 (230.8438, 601.9601) -> (230.8438, 602.2886)
  line L724 (230.8438, 602.2886) -> (233.1063, 602.2886)
  line L725 (233.1063, 602.2886) -> (233.1063, 601.9601)
  line L726 (235.4504, 600.3596) -> (233.9634, 600.3596)
  line L727 (233.9634, 600.3596) -> (233.9634, 600.6708)
  line L728 (233.9634, 600.6708) -> (234.5167, 600.6708)
  line L729 (234.5167, 600.6708) -> (234.5167, 602.7135)
  line L730 (234.5167, 602.7135) -> (233.9634, 602.7135)
  line L731 (233.9634, 602.7135) -> (233.9634, 602.9926)
  spline S685 degree 2 poles (233.9634, 602.9926) (234.2771, 602.9926) (234.5735, 603.1704) (234.5933, 603.4174) knots 0 0 0 1 2 2 2
  line L732 (234.5933, 603.4174) -> (234.9094, 603.4174)
  line L733 (234.9094, 603.4174) -> (234.9094, 600.6708)
  line L734 (234.9094, 600.6708) -> (235.4504, 600.6708)
  line L735 (235.4504, 600.6708) -> (235.4504, 600.3596)
  spline S686 degree 2 poles (237.8586, 601.3278) (237.8586, 601.108) (237.7178, 600.7325) (237.5894, 600.5942) knots 0 0 0 1 2 2 2
  spline S687 degree 2 poles (237.5894, 600.5942) (237.461, 600.4559) (237.0781, 600.2953) (236.841, 600.2953) knots 0 0 0 1 2 2 2
  spline S688 degree 2 poles (236.841, 600.2953) (236.6236, 600.2953) (236.1988, 600.3917) (236.0432, 600.4682) knots 0 0 0 1 2 2 2
  line L736 (236.0432, 600.4682) -> (236.0432, 600.9005)
  line L737 (236.0432, 600.9005) -> (236.0728, 600.9005)
  spline S689 degree 2 poles (236.0728, 600.9005) (236.1197, 600.8659) (236.2951, 600.777) (236.4013, 600.7375) knots 0 0 0 1 2 2 2
  spline S690 degree 2 poles (236.4013, 600.7375) (236.5224, 600.6955) (236.7224, 600.6486) (236.8484, 600.6486) knots 0 0 0 1 2 2 2
  spline S691 degree 2 poles (236.8484, 600.6486) (236.9719, 600.6486) (237.2041, 600.7375) (237.2881, 600.8338) knots 0 0 0 1 2 2 2
  spline S692 degree 2 poles (237.2881, 600.8338) (237.3646, 600.9252) (237.4437, 601.1673) (237.4437, 601.3303) knots 0 0 0 1 2 2 2
  spline S693 degree 2 poles (237.4437, 601.3303) (237.4437, 601.4933) (237.3548, 601.7008) (237.2708, 601.7699) knots 0 0 0 1 2 2 2
  spline S694 degree 2 poles (237.2708, 601.7699) (237.1843, 601.8465) (236.9274, 601.9107) (236.7718, 601.9107) knots 0 0 0 1 2 2 2
  spline S695 degree 2 poles (236.7718, 601.9107) (236.6039, 601.9107) (236.2704, 601.8589) (236.1691, 601.8366) knots 0 0 0 1 2 2 2
  line L738 (236.1691, 601.8366) -> (236.1691, 603.4076)
  line L739 (236.1691, 603.4076) -> (237.8414, 603.4076)
  line L740 (237.8414, 603.4076) -> (237.8414, 603.0494)
  line L741 (237.8414, 603.0494) -> (236.5619, 603.0494)
  line L742 (236.5619, 603.0494) -> (236.5619, 602.2368)
  spline S696 degree 2 poles (236.5619, 602.2368) (236.636, 602.2467) (236.7792, 602.2541) (236.8385, 602.2541) knots 0 0 0 1 2 2 2
  spline S697 degree 2 poles (236.8385, 602.2541) (237.0732, 602.2541) (237.3967, 602.1775) (237.5449, 602.0639) knots 0 0 0 1 2 2 2
  spline S698 degree 2 poles (237.5449, 602.0639) (237.6956, 601.9503) (237.8586, 601.6045) (237.8586, 601.3278) knots 0 0 0 1 2 2 2
  line L743 (240.2595, 601.4069) -> (239.8964, 601.4069)
  line L744 (239.8964, 601.4069) -> (239.8964, 600.3596)
  line L745 (239.8964, 600.3596) -> (239.5037, 600.3596)
  line L746 (239.5037, 600.3596) -> (239.5037, 601.4069)
  line L747 (239.5037, 601.4069) -> (238.1575, 601.4069)
  line L748 (238.1575, 601.4069) -> (238.1575, 601.8366)
  line L749 (238.1575, 601.8366) -> (239.521, 603.4076)
  line L750 (239.521, 603.4076) -> (239.8964, 603.4076)
  line L751 (239.8964, 603.4076) -> (239.8964, 601.7354)
  line L752 (239.8964, 601.7354) -> (240.2595, 601.7354)
  line L753 (240.2595, 601.7354) -> (240.2595, 601.4069)
  line L754 (239.5037, 601.7354) -> (239.5037, 602.9259)
  line L755 (239.5037, 602.9259) -> (238.4786, 601.7354)
  line L756 (238.4786, 601.7354) -> (239.5037, 601.7354)
  spline S699 degree 2 poles (242.5122, 601.3476) (242.5122, 601.1129) (242.3565, 600.7152) (242.2256, 600.5819) knots 0 0 0 1 2 2 2
  spline S700 degree 2 poles (242.2256, 600.5819) (242.0898, 600.4411) (241.7489, 600.2953) (241.5439, 600.2953) knots 0 0 0 1 2 2 2
  spline S701 degree 2 poles (241.5439, 600.2953) (241.3389, 600.2953) (241.0005, 600.4337) (240.8721, 600.572) knots 0 0 0 1 2 2 2
  spline S702 degree 2 poles (240.8721, 600.572) (240.714, 600.7375) (240.5361, 601.2932) (240.5361, 601.6983) knots 0 0 0 1 2 2 2
  spline S703 degree 2 poles (240.5361, 601.6983) (240.5361, 602.096) (240.6992, 602.7357) (240.8696, 602.9728) knots 0 0 0 1 2 2 2
  spline S704 degree 2 poles (240.8696, 602.9728) (241.0351, 603.205) (241.5587, 603.4644) (241.9021, 603.4644) knots 0 0 0 1 2 2 2
  spline S705 degree 2 poles (241.9021, 603.4644) (242.0033, 603.4644) (242.1812, 603.4446) (242.2479, 603.4224) knots 0 0 0 1 2 2 2
  line L757 (242.2479, 603.4224) -> (242.2479, 603.0297)
  line L758 (242.2479, 603.0297) -> (242.2306, 603.0297)
  spline S706 degree 2 poles (242.2306, 603.0297) (242.1738, 603.0593) (241.9663, 603.1112) (241.8477, 603.1112) knots 0 0 0 1 2 2 2
  spline S707 degree 2 poles (241.8477, 603.1112) (241.4673, 603.1112) (241.0005, 602.5974) (240.956, 602.0935) knots 0 0 0 1 2 2 2
  spline S708 degree 2 poles (240.956, 602.0935) (241.1018, 602.1948) (241.4081, 602.3059) (241.5908, 602.3059) knots 0 0 0 1 2 2 2
  spline S709 degree 2 poles (241.5908, 602.3059) (241.7687, 602.3059) (242.0354, 602.2343) (242.1812, 602.1256) knots 0 0 0 1 2 2 2
  spline S710 degree 2 poles (242.1812, 602.1256) (242.3491, 601.9997) (242.5122, 601.6094) (242.5122, 601.3476) knots 0 0 0 1 2 2 2
  spline S711 degree 2 poles (242.0972, 601.3303) (242.0972, 601.518) (241.9984, 601.7724) (241.8897, 601.8613) knots 0 0 0 1 2 2 2
  spline S712 degree 2 poles (241.8897, 601.8613) (241.8082, 601.9256) (241.6057, 601.9675) (241.4994, 601.9675) knots 0 0 0 1 2 2 2
  spline S713 degree 2 poles (241.4994, 601.9675) (241.3562, 601.9675) (241.087, 601.8811) (240.956, 601.7996) knots 0 0 0 1 2 2 2
  spline S714 degree 2 poles (240.956, 601.7996) (240.9536, 601.7551) (240.9486, 601.6711) (240.9486, 601.6069) knots 0 0 0 1 2 2 2
  spline S715 degree 2 poles (240.9486, 601.6069) (240.9486, 601.2908) (241.0721, 600.903) (241.166, 600.8017) knots 0 0 0 1 2 2 2
  spline S716 degree 2 poles (241.166, 600.8017) (241.2524, 600.7054) (241.4402, 600.6288) (241.5464, 600.6288) knots 0 0 0 1 2 2 2
  spline S717 degree 2 poles (241.5464, 600.6288) (241.7934, 600.6288) (242.0972, 600.9795) (242.0972, 601.3303) knots 0 0 0 1 2 2 2
  line L759 (244.5993, 600.3596) -> (243.1124, 600.3596)
  line L760 (243.1124, 600.3596) -> (243.1124, 600.6708)
  line L761 (243.1124, 600.6708) -> (243.6656, 600.6708)
  line L762 (243.6656, 600.6708) -> (243.6656, 602.7135)
  line L763 (243.6656, 602.7135) -> (243.1124, 602.7135)
  line L764 (243.1124, 602.7135) -> (243.1124, 602.9926)
  spline S718 degree 2 poles (243.1124, 602.9926) (243.4261, 602.9926) (243.7225, 603.1704) (243.7422, 603.4174) knots 0 0 0 1 2 2 2
  line L765 (243.7422, 603.4174) -> (244.0584, 603.4174)
  line L766 (244.0584, 603.4174) -> (244.0584, 600.6708)
  line L767 (244.0584, 600.6708) -> (244.5993, 600.6708)
  line L768 (244.5993, 600.6708) -> (244.5993, 600.3596)
  line L769 (247.1212, 601.4069) -> (246.7581, 601.4069)
  line L770 (246.7581, 601.4069) -> (246.7581, 600.3596)
  line L771 (246.7581, 600.3596) -> (246.3654, 600.3596)
  line L772 (246.3654, 600.3596) -> (246.3654, 601.4069)
  line L773 (246.3654, 601.4069) -> (245.0192, 601.4069)
  line L774 (245.0192, 601.4069) -> (245.0192, 601.8366)
  line L775 (245.0192, 601.8366) -> (246.3827, 603.4076)
  line L776 (246.3827, 603.4076) -> (246.7581, 603.4076)
  line L777 (246.7581, 603.4076) -> (246.7581, 601.7354)
  line L778 (246.7581, 601.7354) -> (247.1212, 601.7354)
  line L779 (247.1212, 601.7354) -> (247.1212, 601.4069)
  line L780 (246.3654, 601.7354) -> (246.3654, 602.9259)
  line L781 (246.3654, 602.9259) -> (245.3403, 601.7354)
  line L782 (245.3403, 601.7354) -> (246.3654, 601.7354)
  spline S719 degree 2 poles (248.2698, 603.1186) (248.1586, 603.1186) (247.9388, 603.0642) (247.8326, 603.0222) knots 0 0 0 1 2 2 2
  spline S720 degree 2 poles (247.8326, 603.0222) (247.7338, 602.9803) (247.588, 602.8913) (247.5312, 602.8518) knots 0 0 0 1 2 2 2
  line L783 (247.5312, 602.8518) -> (247.5065, 602.8518)
  line L784 (247.5065, 602.8518) -> (247.5065, 603.2841)
  spline S721 degree 2 poles (247.5065, 603.2841) (247.6399, 603.3557) (248.0969, 603.4718) (248.3019, 603.4718) knots 0 0 0 1 2 2 2
  spline S722 degree 2 poles (248.3019, 603.4718) (248.5094, 603.4718) (248.8181, 603.3878) (248.9441, 603.2989) knots 0 0 0 1 2 2 2
  spline S723 degree 2 poles (248.9441, 603.2989) (249.0775, 603.2026) (249.2158, 602.9234) (249.2158, 602.7357) knots 0 0 0 1 2 2 2
  spline S724 degree 2 poles (249.2158, 602.7357) (249.2158, 602.4838) (248.8848, 602.1034) (248.6526, 602.054) knots 0 0 0 1 2 2 2
  line L785 (248.6526, 602.054) -> (248.6526, 602.0244)
  spline S725 degree 2 poles (248.6526, 602.0244) (248.7489, 602.0046) (248.9688, 601.9157) (249.0626, 601.8268) knots 0 0 0 1 2 2 2
  spline S726 degree 2 poles (249.0626, 601.8268) (249.1565, 601.7403) (249.2751, 601.4637) (249.2751, 601.2636) knots 0 0 0 1 2 2 2
  spline S727 degree 2 poles (249.2751, 601.2636) (249.2751, 601.0586) (249.1343, 600.7103) (249.0058, 600.5769) knots 0 0 0 1 2 2 2
  spline S728 degree 2 poles (249.0058, 600.5769) (248.8724, 600.4386) (248.4945, 600.2953) (248.2549, 600.2953) knots 0 0 0 1 2 2 2
  spline S729 degree 2 poles (248.2549, 600.2953) (248.0252, 600.2953) (247.5757, 600.4065) (247.4225, 600.4831) knots 0 0 0 1 2 2 2
  line L786 (247.4225, 600.4831) -> (247.4225, 600.9153)
  line L787 (247.4225, 600.9153) -> (247.4522, 600.9153)
  spline S730 degree 2 poles (247.4522, 600.9153) (247.5806, 600.8215) (248.0153, 600.6486) (248.2302, 600.6486) knots 0 0 0 1 2 2 2
  spline S731 degree 2 poles (248.2302, 600.6486) (248.3562, 600.6486) (248.6082, 600.7276) (248.6921, 600.819) knots 0 0 0 1 2 2 2
  spline S732 degree 2 poles (248.6921, 600.819) (248.7736, 600.9104) (248.8601, 601.1277) (248.8601, 601.2932) knots 0 0 0 1 2 2 2
  spline S733 degree 2 poles (248.8601, 601.2932) (248.8601, 601.4587) (248.7638, 601.6736) (248.6773, 601.7354) knots 0 0 0 1 2 2 2
  spline S734 degree 2 poles (248.6773, 601.7354) (248.5909, 601.7971) (248.3562, 601.844) (248.2179, 601.844) knots 0 0 0 1 2 2 2
  line L788 (248.2179, 601.844) -> (248.045, 601.844)
  line L789 (248.045, 601.844) -> (248.045, 602.1824)
  line L790 (248.045, 602.1824) -> (248.1808, 602.1824)
  spline S735 degree 2 poles (248.1808, 602.1824) (248.455, 602.1824) (248.8008, 602.4443) (248.8008, 602.6937) knots 0 0 0 1 2 2 2
  spline S736 degree 2 poles (248.8008, 602.6937) (248.8008, 602.8098) (248.7119, 602.9753) (248.6403, 603.0247) knots 0 0 0 1 2 2 2
  spline S737 degree 2 poles (248.6403, 603.0247) (248.5637, 603.0766) (248.376, 603.1186) (248.2698, 603.1186) knots 0 0 0 1 2 2 2
  spline S738 degree 2 poles (250.557, 603.1186) (250.4458, 603.1186) (250.226, 603.0642) (250.1198, 603.0222) knots 0 0 0 1 2 2 2
  spline S739 degree 2 poles (250.1198, 603.0222) (250.021, 602.9803) (249.8753, 602.8913) (249.8185, 602.8518) knots 0 0 0 1 2 2 2
  line L791 (249.8185, 602.8518) -> (249.7938, 602.8518)
  line L792 (249.7938, 602.8518) -> (249.7938, 603.2841)
  spline S740 degree 2 poles (249.7938, 603.2841) (249.9271, 603.3557) (250.3841, 603.4718) (250.5891, 603.4718) knots 0 0 0 1 2 2 2
  spline S741 degree 2 poles (250.5891, 603.4718) (250.7966, 603.4718) (251.1053, 603.3878) (251.2313, 603.2989) knots 0 0 0 1 2 2 2
  spline S742 degree 2 poles (251.2313, 603.2989) (251.3647, 603.2026) (251.503, 602.9234) (251.503, 602.7357) knots 0 0 0 1 2 2 2
  spline S743 degree 2 poles (251.503, 602.7357) (251.503, 602.4838) (251.172, 602.1034) (250.9398, 602.054) knots 0 0 0 1 2 2 2
  line L793 (250.9398, 602.054) -> (250.9398, 602.0244)
  spline S744 degree 2 poles (250.9398, 602.0244) (251.0362, 602.0046) (251.256, 601.9157) (251.3499, 601.8268) knots 0 0 0 1 2 2 2
  spline S745 degree 2 poles (251.3499, 601.8268) (251.4437, 601.7403) (251.5623, 601.4637) (251.5623, 601.2636) knots 0 0 0 1 2 2 2
  spline S746 degree 2 poles (251.5623, 601.2636) (251.5623, 601.0586) (251.4215, 600.7103) (251.2931, 600.5769) knots 0 0 0 1 2 2 2
  spline S747 degree 2 poles (251.2931, 600.5769) (251.1597, 600.4386) (250.7818, 600.2953) (250.5422, 600.2953) knots 0 0 0 1 2 2 2
  spline S748 degree 2 poles (250.5422, 600.2953) (250.3125, 600.2953) (249.8629, 600.4065) (249.7098, 600.4831) knots 0 0 0 1 2 2 2
  line L794 (249.7098, 600.4831) -> (249.7098, 600.9153)
  line L795 (249.7098, 600.9153) -> (249.7394, 600.9153)
  spline S749 degree 2 poles (249.7394, 600.9153) (249.8679, 600.8215) (250.3026, 600.6486) (250.5175, 600.6486) knots 0 0 0 1 2 2 2
  spline S750 degree 2 poles (250.5175, 600.6486) (250.6434, 600.6486) (250.8954, 600.7276) (250.9794, 600.819) knots 0 0 0 1 2 2 2
  spline S751 degree 2 poles (250.9794, 600.819) (251.0609, 600.9104) (251.1473, 601.1277) (251.1473, 601.2932) knots 0 0 0 1 2 2 2
  spline S752 degree 2 poles (251.1473, 601.2932) (251.1473, 601.4587) (251.051, 601.6736) (250.9645, 601.7354) knots 0 0 0 1 2 2 2
  spline S753 degree 2 poles (250.9645, 601.7354) (250.8781, 601.7971) (250.6434, 601.844) (250.5051, 601.844) knots 0 0 0 1 2 2 2
  line L796 (250.5051, 601.844) -> (250.3322, 601.844)
  line L797 (250.3322, 601.844) -> (250.3322, 602.1824)
  line L798 (250.3322, 602.1824) -> (250.4681, 602.1824)
  spline S754 degree 2 poles (250.4681, 602.1824) (250.7422, 602.1824) (251.088, 602.4443) (251.088, 602.6937) knots 0 0 0 1 2 2 2
  spline S755 degree 2 poles (251.088, 602.6937) (251.088, 602.8098) (250.9991, 602.9753) (250.9275, 603.0247) knots 0 0 0 1 2 2 2
  spline S756 degree 2 poles (250.9275, 603.0247) (250.8509, 603.0766) (250.6632, 603.1186) (250.557, 603.1186) knots 0 0 0 1 2 2 2
  line L799 (253.7483, 600.3596) -> (252.2613, 600.3596)
  line L800 (252.2613, 600.3596) -> (252.2613, 600.6708)
  line L801 (252.2613, 600.6708) -> (252.8146, 600.6708)
  line L802 (252.8146, 600.6708) -> (252.8146, 602.7135)
  line L803 (252.8146, 602.7135) -> (252.2613, 602.7135)
  line L804 (252.2613, 602.7135) -> (252.2613, 602.9926)
  spline S757 degree 2 poles (252.2613, 602.9926) (252.575, 602.9926) (252.8714, 603.1704) (252.8912, 603.4174) knots 0 0 0 1 2 2 2
  line L805 (252.8912, 603.4174) -> (253.2073, 603.4174)
  line L806 (253.2073, 603.4174) -> (253.2073, 600.6708)
  line L807 (253.2073, 600.6708) -> (253.7483, 600.6708)
  line L808 (253.7483, 600.6708) -> (253.7483, 600.3596)
  line L809 (256.1886, 600.3596) -> (254.3089, 600.3596)
  line L810 (254.3089, 600.3596) -> (254.3089, 600.7918)
  spline S758 degree 2 poles (254.3089, 600.7918) (254.5115, 600.982) (254.8721, 601.3352) (255.045, 601.5254) knots 0 0 0 1 2 2 2
  spline S759 degree 2 poles (255.045, 601.5254) (255.3933, 601.9083) (255.6477, 602.3677) (255.6477, 602.6122) knots 0 0 0 1 2 2 2
  spline S760 degree 2 poles (255.6477, 602.6122) (255.6477, 602.7407) (255.5687, 602.9333) (255.497, 602.9951) knots 0 0 0 1 2 2 2
  spline S761 degree 2 poles (255.497, 602.9951) (255.4254, 603.0568) (255.2377, 603.1186) (255.1241, 603.1186) knots 0 0 0 1 2 2 2
  spline S762 degree 2 poles (255.1241, 603.1186) (255.0154, 603.1186) (254.7931, 603.0642) (254.6918, 603.0222) knots 0 0 0 1 2 2 2